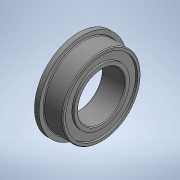
# Autodesk Inventor part: FL676ZZ
Saved by Autodesk Inventor 2022 (Build 260153000, 153)
## iProperties
Category: PARTsolutions
Company: MISUMI
Part Number: FL676ZZ
Material: 一般
Catalog Web Link: www.cadenas.de
Description: FL6 _ _ ZZ, FL6 _ _ AZZ, SFL6 _ _ ZZ, SFL6 _ _ AZZ, MFL1 _ _ ZZ, SMFL1 _ _ ZZ-Flanged Ball Bearings (Small Diameter, Deep Groove) - Double Shield Type
Vendor: MISUMI
Document SubType Name: Modeling
Designer: partserver
Manufacturer: MISUMI
Mass: 0.147381 g
Surface Area: 3.26668 cm^2
Volume: 0.147381 cm^3
Density: 1 g/cm^3
Appearance: PSOLRGB-175-175-175
PSOL_IDENT_0: {$CADENAS_DATA\23d-libs\misumi\metric\12_bearing_holders\sfl608zz.prj},229 {VTYP=3D},{NB=FL676ZZ},{L
PSOL_IDENT_1: INA=FL676ZZ},{NN=FL6 _ _ ZZ, FL6 _ _ AZZ, SFL6 _ _ ZZ, SFL6 _ _ AZZ, MFL1 _ _ ZZ, SMFL1 _ _ ZZ},{DAT
PSOL_IDENT_2: E=09.09.2019 15:26:56},{GEOMDATE=16.08.2017 04:27:24},{VERSION=},{LINEID=100},{WBVAR=MAT},{WBNUMERIC=
PSOL_IDENT_3: }  {NB=FL676ZZ},{LINA=FL676ZZ},{KT=DUMMY},{PN=FL676ZZ},{MAT=},{MAT1= '', '52100 Bearing Steel', 'S',
PSOL_IDENT_4: '440C Stainless Steel'},{BN=676ZZ},{DD=6.0},{AA=2.4600},{BB=0.4000},{C1=0.5500},{D=10},{B=3.0},{D1=
PSOL_IDENT_5: 11.2},{C=0.6},{RR=0.10},{CR=465},{COR=196},{CRS=465},{CRSS=422},{CORS=196},{CORSS=174},{DS=6.60},{R=
PSOL_IDENT_6: 0.10},{MASS=0.74},{MAT11=1},{MMMM=}
NB: FL676ZZ
NN: FL6 _ _ ZZ, FL6 _ _ AZZ, SFL6 _ _ ZZ, SFL6 _ _ AZZ, MFL1 _ _ ZZ, SMFL1 _ _ ZZ
NT: Flanged Ball Bearings (Small Diameter, Deep Groove) - Double Shield Type
NBSYN: $PN.
LINA: FL676ZZ
CATALOG: Misumi
PN: FL676ZZ
MAT: 52100 Bearing Steel
BN: 676ZZ
DD: 6
D: 10
B: 3
D1: 11.2
C: 0.6
RR: 0.1
CR: 465
COR: 196
DS: 6.6
R: 0.1
MASS: 0.74
SUPPLIER: MISUMI
ARTICLENO: FL676ZZ
BOMINFO: FL676ZZ
CREATOR: CADENAS GmbH
Title: FL676ZZ
Author: Cadenas PARTsolutions
Comments: Flanged Ball Bearings (Small Diameter, Deep Groove) - Double Shield Type
Autodesk Inventor part; units mm, degrees
sketch "Sketch_1" plane through (0, 0, 0) normal (0, 0, 1) x (1, 0, 0)
  line L0 (10, 0) -> (-10, 0)
  arc A0 (0, 3.1) -> (0.1, 3) centre (0.1, 3.1) ccw
  line L1 (0.1, 3) -> (2.9, 3)
  arc A1 (2.9, 3) -> (3, 3.1) centre (2.9, 3.1) ccw
  line L2 (3, 3.1) -> (3, 3.55)
  line L3 (3, 3.55) -> (2.73, 3.55)
  line L4 (2.73, 3.55) -> (2.73, 4.6)
  line L5 (2.73, 4.6) -> (3, 4.6)
  line L6 (3, 4.6) -> (3, 5.6)
  line L7 (3, 5.6) -> (2.4, 5.6)
  line L8 (2.4, 5.6) -> (2.4, 5.1)
  arc A2 (2.3, 5) -> (2.4, 5.1) centre (2.4, 5) ccw
  line L9 (2.3, 5) -> (0.1, 5)
  arc A3 (0.1, 5) -> (0, 4.9) centre (0.1, 4.9) ccw
  line L10 (0, 4.9) -> (0, 4.6)
  line L11 (0, 4.6) -> (0.27, 4.6)
  line L12 (0.27, 4.6) -> (0.27, 3.55)
  line L13 (0.27, 3.55) -> (0, 3.55)
  line L14 (0, 3.55) -> (0, 3.1)
  constraints: 30 end point, 8 point on circle, 4 centre point
revolve "Revolution1" add sketch "Sketch_1" angle 360 about axis through (10, 0, 0) along (1, 0, 0)
ref_plane "to_housing_XY" through (0, 0, 0) normal (1, 0, 0) x (0, 0, -1)
ref_plane "to_housing_YZ" through (0, 0, 0) normal (0, 0, -1) x (0, 1, 0)
ref_plane "to_housing_ZX" through (0, 0, 0) normal (0, 1, 0) x (1, 0, 0)
body "Solid1"
